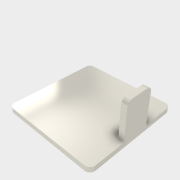
# Autodesk Inventor part: PWTR-0082
Saved by Autodesk Inventor 2021.1 (Build 251245000, 245)
## iProperties
Created: 2020-08-28
Part Number: PWTR-0082
Material: Aluminum 6061
Document SubType Name: Modeling
Designer: alid
Density: 2.7 g/cm^3
Appearance: Titanium - Polished
Author: alid
Autodesk Inventor part; units mm, degrees
ref_plane "YZ Plane" through (0, 0, 0) normal (1, 0, 0) x (0, 1, 0)
ref_plane "XZ Plane" through (0, 0, 0) normal (0, 1, 0) x (-1, 0, 0)
ref_plane "XY Plane" through (0, 0, 0) normal (0, 0, 1) x (1, 0, 0)
sketch "Sketch1" plane through (0, 0, 0) normal (0, 0, 1) x (1, 0, 0)
  line L0 (-90, 90) -> (90, 90)
  line L1 (90, 90) -> (90, -90)
  line L2 (90, -90) -> (-90, -90)
  line L3 (-90, -90) -> (-90, 90)
  line L4 (90, 40) -> (165, 40)
  line L5 (165, 40) -> (165, -40)
  line L6 (165, -40) -> (90, -40)
  line L7 (90, -40) -> (90, 40)
  point P0 (0, 0)
  point P1 (-90, 0)
  point P2 (165, 0)
  point P3 (90, 0)
  point P4 (90, -40)
  dimension "d0" = 90
  dimension "d1" = 180
  dimension "d2" = 180
  dimension "d29" = 75
  dimension "d30" = 80
  constraints: 16 end point, 4 parallel, 3 midpoint, 2 horizontal, 2 horizontal alignment, 2 perpendicular, 1 point on line
  measures "d0" distance from line of point (0, 0) L3
  measures "d1" distance of L0.start L0.end
  measures "d2" distance of L2.end L0.start
  measures "d29" distance of L5.end L6.end
  measures "d30" distance of L4.end L5.end
extrude "Extrusion1" add sketch "Sketch1" along normal blind 10 contours L0 L1 L2 L3
sketch "Sketch3" plane through (-90, -90, 0) normal (0, -1, 0) x (1, 0, 0)
  line L0 (0, 0) -> (180, 0) projected
  line L1 (180, 0) -> (180, 10) projected
  line L2 (0, 10) -> (180, 10) projected
  line L3 (0, 0) -> (0, 10) projected
  line L4 (65, 10) -> (65, 80)
  line L5 (65, 80) -> (115, 80)
  line L6 (115, 80) -> (115, 10)
  line L7 (0, 10) -> (180, 10) projected
  point P0 (90, 0)
  point P1 (90, 80)
  point P2 (90, 10)
  dimension "d22" = 70
  dimension "d23" = 50
  constraints: 6 end point, 3 perpendicular, 2 midpoint, 2 point on line, 1 vertical alignment
  measures "d22" distance of L4.start L4.end
  measures "d23" distance of L4.end L5.end
extrude "Extrusion4" add sketch "Sketch3" against normal blind 10 contours L4 L5 L6 L2
fillet "Fillet4" radius 10 6 edges at (-90, 90, 5) (90, 90, 5) (-90, -90, 5) (90, -90, 5) (-25, -85, 80) (25, -85, 80)
sketch "Sketch4" plane through (90, -40, 0) normal (0, -1, 0) x (1, 0, 0)
  line L0 (0, 0) -> (75, 0) projected
  line L1 (75, 0) -> (75, 10) projected
  line L2 (0, 10) -> (75, 10) projected
  line L3 (0, 0) -> (0, 10) projected
  line L4 (75, 10) -> (62.895, 55.1764)
  arc A0 (62.895, 55.1764) -> (27.3654, 61.7133) centre (43.5765, 50) ccw
  line L5 (0, 10) -> (-10, 10)
  line L6 (-10, 10) -> (27.3654, 61.7133)
  point P0 (-90, 0)
  dimension "d31" = 75
  dimension "d32" = 20
  dimension "d33" = 40
  dimension "d36" = 10
  constraints: 6 end point, 2 point on circle, 2 tangent, 1 centre point, 1 horizontal
  measures "d31" angle of L2 L4
  measures "d32" radius of A0
  measures "d33" distance from line of L2 A0.centre
  measures "d36" distance of L2.start L5.end
equation "\"d0\" = 0.5 * d1"
equation "\"d24\" = d3"
equation "\"d3\" = 10"
body "Solid1"
